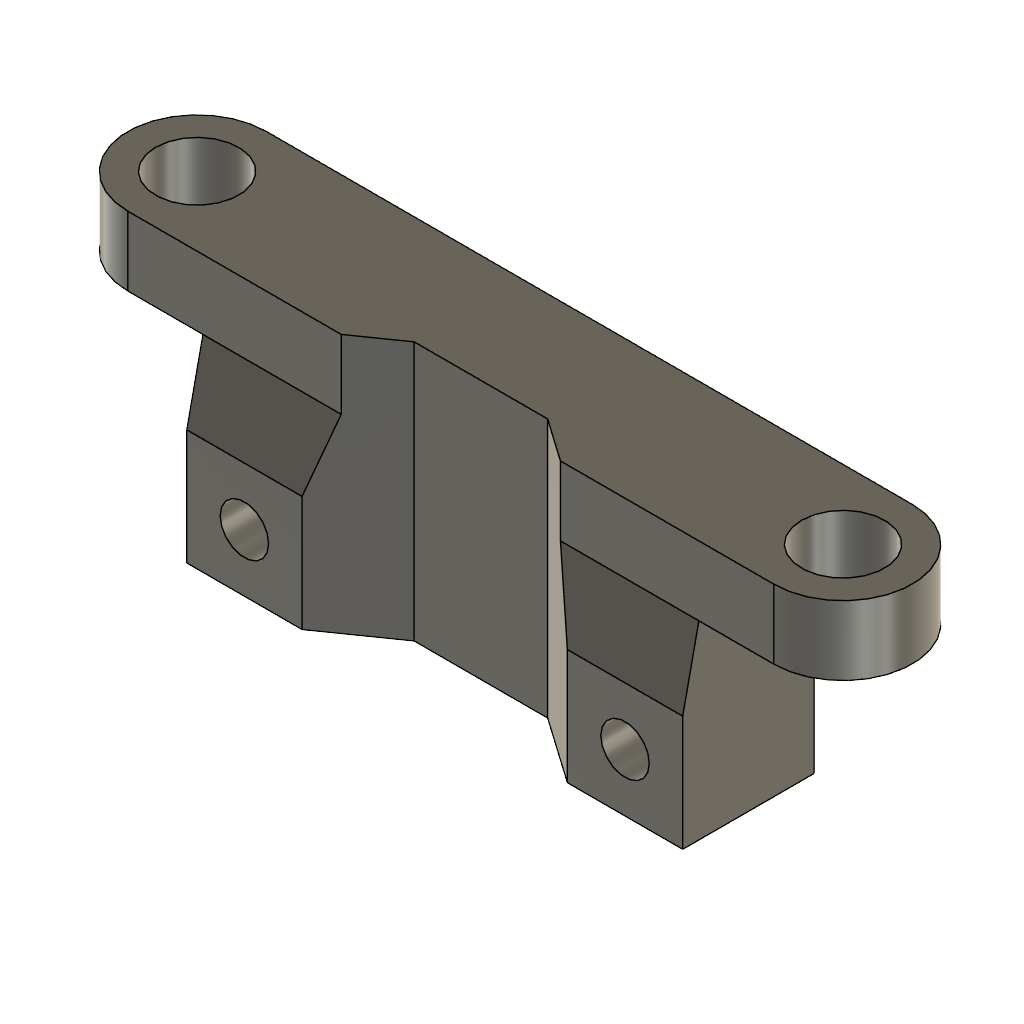
USB Halter (Autodesk Fusion 360 design; units mm, degrees)
Autodesk Fusion 360 part; units mm, degrees
sketch "Skizze1" plane through (0, 0, 0) normal (0, 0, 1) x (1, 0, 0)
  circle A0 centre (0, 0) radius 1.8
  circle A1 centre (-28, 0) radius 1.8
  line L0 (-28, 0) -> (0, 0) construction
  line L1 (-28, 3) -> (0, 3)
  line L2 (-28, -3) -> (0, -3)
  arc A2 (-28, 3) -> (-28, -3) centre (-28, 0) ccw
  arc A3 (0, -3) -> (0, 3) centre (0, 0) ccw
  dimension "d1" = 3.6
  dimension "d2" = 28
  dimension "d3" = 6
  constraint coincident A0.centre L0.end
  constraint coincident A1.centre L0.start
  constraint horizontal L0
  constraint equal A0 A1
  constraint concentric A1 A2
  constraint equal A2 A3
  constraint horizontal L1
  constraint parallel L0 L2
  constraint tangent L1 A3
  constraint tangent L2 A3
  measures "d1" diameter of A1
  measures "d2" distance of A0.centre A1.centre
  measures "d3" diameter of A2
extrude "Extrusion1" add sketch "Skizze1" along normal blind 3
sketch "Skizze2" plane through (0, 0, 0) normal (0, 0, 1) x (-1, 0, 0)
  circle A0 centre (0, 0) radius 1.8
  circle A1 centre (28, 0) radius 1.8
  arc A2 (28, -3) -> (28, 3) centre (28, 0) ccw
  line L0 (28, 3) -> (0, 3)
  arc A3 (0, 3) -> (0, -3) centre (0, 0) ccw
  line L1 (0, -3) -> (28, -3)
  line L2 (24.75, -3) -> (3.25, -3)
  line L3 (3.25, -3) -> (3.25, 3.7)
  line L4 (3.25, 3.7) -> (24.75, 3.7)
  line L5 (24.75, 3.7) -> (24.75, -3)
  circle A4 centre (0, 0) radius 1.8
  circle A5 centre (28, 0) radius 1.8
  arc A6 (28, -3) -> (28, 3) centre (28, 0) ccw
  line L6 (28, -3) -> (0, -3)
  arc A7 (0, 3) -> (0, -3) centre (0, 0) ccw
  line L7 (0, 3) -> (28, 3)
  line L8 (28, 0) -> (0, 0) construction
  line L9 (14, 0) -> (14, 18.5057) construction
  dimension "d9" = 0.7
  dimension "d10" = 21.5
  constraint horizontal L2
  constraint vertical L3
  constraint horizontal L4
  constraint vertical L5
  constraint coincident L1 L2.start
  constraint coincident A1.centre A2.centre
  constraint coincident A0.centre A3.centre
  constraint midpoint L8 L9.start
  constraint perpendicular L8 L9
  constraint symmetric L3 L5 L9
  measures "d9" distance of L0 L4
  measures "d10" distance of L3.end L4.end
extrude "Extrusion2" add sketch "Skizze2" against normal blind 8.23 contours L0 L1 L2 L3 L5 L6 L7 | L0 L3 L4 L5 L7
sketch "Skizze3" plane through (0, 3, 0) normal (0, 1, 0) x (-1, 0, 0)
  line L0 (24.75, 0) -> (28, 0)
  line L1 (28, 0) -> (28, 3)
  line L2 (28, 3) -> (0, 3)
  line L3 (0, 3) -> (0, 0)
  line L4 (0, 0) -> (3.25, 0)
  line L5 (3.25, 0) -> (3.25, -8.23)
  line L6 (3.25, -8.23) -> (24.75, -8.23)
  line L7 (24.75, -8.23) -> (24.75, 0)
  circle A0 centre (22.25, -5.73) radius 1.05
  circle A1 centre (5.75, -5.73) radius 1.05
  line L8 (24.75, -5.73) -> (3.25, -5.73) construction
  dimension "d11" = 2.1
  dimension "d13" = 2.5
  dimension "d14" = 2.5
  dimension "d15" = 2.5
  constraint coincident L7 L8.start
  constraint coincident L5 L8.end
  constraint perpendicular L5 L8
  constraint coincident A1.centre L8
  constraint coincident A0.centre L8
  constraint equal A0 A1
  measures "d11" diameter of A0
  measures "d13" distance of L7 A0.centre
  measures "d14" distance of L5 A1.centre
  measures "d15" distance of L6 L8
extrude "Extrusion3" cut sketch "Skizze3" against normal up to surface (6.7 mm away) contours A0 | A1
chamfer "Fase1" distance 1 angle 45 3 edges at (-24.75, 3, -4.115) (-14, 3, -8.23) (-3.25, 3, -4.115)
sketch "Skizze4" plane through (-24.75, 0, 0) normal (-1, 0, 0) x (0, -1, 0)
  line L0 (-2, 0) -> (-2, -8.23)
  line L1 (-2, -8.23) -> (3.7, -8.23)
  line L2 (3.7, -8.23) -> (3.7, 0)
  line L3 (3.7, 0) -> (3, 0)
  line L4 (3, 0) -> (-2, 0)
  line L5 (3.7, -4.68) -> (3.7, -6.78)
  line L6 (3.7, -4.68) -> (3.7, -6.78)
  line L7 (3.7, 0) -> (3.7, -8.23)
  line L8 (3.7, -8.23) -> (3.7, 0)
  line L9 (3, 0) -> (3, 3)
  line L10 (3, 3) -> (3, 0)
  line L11 (3, 0) -> (3.7, 0)
  line L12 (3.7, 0) -> (3, 0)
  line L13 (3.7, -3.23) -> (3.7, 0)
  line L14 (3, 0) -> (3.7, -3.23)
  dimension "d29" = 5
  constraint coincident L8 L13.start
  constraint coincident L2.end L3.start
  constraint coincident L3.end L4.start
  measures "d29" distance of L1.end L13.start
extrude "Extrusion4" cut sketch "Skizze4" against normal up to surface (21.5 mm away) contours L2 L3 L7 L8 L11 L12 L13 L14
sketch "Skizze5" plane through (0, 0, -8.23) normal (0, 0, -1) x (1, 0, 0)
  line L0 (-24.75, -2) -> (-3.25, -2)
  line L1 (-3.25, -2) -> (-3.25, 3.7)
  line L2 (-3.25, 3.7) -> (-24.75, 3.7)
  line L3 (-24.75, 3.7) -> (-24.75, -2)
  line L4 (-19.75, 3.7) -> (-16.8937, 1.7)
  line L5 (-16.8937, 1.7) -> (-11.1063, 1.7)
  line L6 (-11.1063, 1.7) -> (-8.25, 3.7)
  line L7 (-14, 3.7) -> (-14, -2) construction
  line L8 (-19.75, 3.7) -> (-8.25, 3.7)
  dimension "d22" = 5
  dimension "d24" = 2
  dimension "d25" = 35
  constraint coincident L2 L4.start
  constraint horizontal L5
  constraint coincident L2 L6.end
  constraint midpoint L2 L7.start
  constraint midpoint L0 L7.end
  constraint symmetric L4.end L5.end L7
  constraint symmetric L4.start L6.end L7
  measures "d22" distance of L2.end L4.start
  measures "d24" distance of L5 L8
  measures "d25" angle of L4 L8
extrude "Extrusion5" cut sketch "Skizze5" against normal up to surface (11.23 mm away) contours L2 L4 L5 L6 L8
equation "d7 = -6.73 mm - 1.5 mm"
equation "d13 = 1 mm + 1.5 mm"
equation "d14 = 1 mm + 1.5 mm"
equation "d15 = 1 mm + 1.5 mm"
equation "d22 = 1 mm + 3 mm + 1 mm"
equation "d29 = 1 mm + 3 mm + 1 mm"
